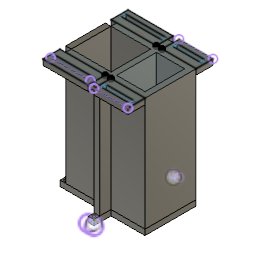
dobot_magician_holder_210mm (Autodesk Fusion 360 design; units mm, degrees)
Autodesk Fusion 360 part; units mm, degrees
note: some values were not read from the file. Chosen so that the rebuilt part matches the saved one: which bodies a step acts on.
sketch "スケッチ1" plane through (0, 0, 0) normal (0, 0, 1) x (1, 0, 0)
  line L0 (5, 75) -> (-5, 75)
  line L1 (-5, 75) -> (-5, -75)
  line L2 (-5, -75) -> (5, -75)
  line L3 (5, -75) -> (5, 75)
  line L4 (5, 75) -> (-5, -75) construction
  line L5 (-5, 75) -> (5, -75) construction
  dimension "d1" = 10
  dimension "d2" = 150
  constraint horizontal L0
  constraint perpendicular L0 L1
  constraint parallel L0 L2
  constraint parallel L1 L3
  constraint coincident L4 origin
  constraint coincident L5 origin
  measures "d1" distance of L1.end L2.end
  measures "d2" distance of L0.end L1.end
sketch "スケッチ2" plane through (0, 0, 0) normal (0, 0, 1) x (1, 0, 0)
  circle A0 centre (0, 70) radius 2.5
  line L0 (5, 75) -> (-5, 75)
  circle A1 centre (0, -70) radius 2.5
  line L1 (-5, -75) -> (5, -75)
  dimension "d3" = 5
  dimension "d4" = 5
  dimension "d5" = 5
  dimension "d6" = 5
  measures "d3" diameter of A0
  measures "d4" distance of A0.centre L0
  measures "d5" diameter of A1
  measures "d6" distance of A1.centre L1
extrude "押し出し1" add sketch "スケッチ1" along normal blind 1 makes body 1
extrude "押し出し2" cut sketch "スケッチ2" along normal blind 2 contours A1 bodies 1
sketch "スケッチ3" plane through (0, 0, 0) normal (0, 0, 1) x (1, 0, 0)
  line L0 (-75, 45) -> (-85, 45)
  line L1 (-85, 45) -> (-85, -45)
  line L2 (-85, -45) -> (-75, -45)
  line L3 (-75, -45) -> (-75, 45)
  line L4 (-75, 45) -> (-85, -45) construction
  line L5 (-85, 45) -> (-75, -45) construction
  circle A0 centre (-80, 40) radius 2.5
  circle A1 centre (-80, -40) radius 2.5
  line L6 (-85, 45) -> (65, 45)
  line L7 (65, 45) -> (65, 35)
  line L8 (65, 35) -> (-85, 35)
  line L9 (-85, 35) -> (-85, 45)
  line L10 (-85, -45) -> (65, -45)
  line L11 (65, -45) -> (65, -35)
  line L12 (65, -35) -> (-85, -35)
  line L13 (-85, -35) -> (-85, -45)
  line L14 (55, 45) -> (65, 45)
  line L15 (65, 45) -> (65, -45)
  line L16 (65, -45) -> (55, -45)
  line L17 (55, -45) -> (55, 45)
  point P0 (-80, 0)
  point P1 (0, 70)
  dimension "d11" = 10
  dimension "d12" = 90
  dimension "d13" = 5
  dimension "d14" = 5
  dimension "d15" = 80
  dimension "d16" = 5
  dimension "d17" = 5
  dimension "d18" = 150
  dimension "d19" = 10
  dimension "d20" = 150
  dimension "d21" = 10
  constraint horizontal L0
  constraint perpendicular L0 L1
  constraint parallel L0 L2
  constraint parallel L1 L3
  constraint coincident L4 P0
  constraint coincident L5 P0
  constraint horizontal L6
  constraint vertical L7
  constraint horizontal L8
  constraint vertical L9
  constraint horizontal L10
  constraint vertical L11
  constraint horizontal L12
  constraint vertical L13
  constraint horizontal L14
  constraint vertical L15
  constraint horizontal L16
  constraint vertical L17
  constraint coincident L6 L14.start
  measures "d11" distance of L1.end L2.end
  measures "d12" distance of L0.end L1.end
  measures "d13" diameter of A0
  measures "d14" diameter of A1
  measures "d15" horizontal distance of A0.centre P1
  measures "d16" distance of L1 A0.centre
  measures "d17" distance of L1 A1.centre
  measures "d18" distance of L0.end L6.end
  measures "d19" distance of L0.end L8.end
  measures "d20" distance of L1.end L10.end
  measures "d21" distance of L1.end L12.end
extrude "押し出し3" add sketch "スケッチ3" along normal blind 1 contours L0 L1 L3 L6 L8 L9 | L3 L6 L8 L17 | L1 L3 L8 L12 | L6 L7 L8 L14 L15 L17 | L3 L10 L12 L17 | L1 L2 L3 L10 L12 L13 | L8 L12 L15 L17 | L10 L11 L12 L15 L16 L17 bodies 1
extrude "押し出し4" cut sketch "スケッチ2" along normal blind 2 contours A0 bodies 1
fillet "フィレット1" radius 1 1 faces at (61.6667, -11.6667, 0) on bodies 1
extrude "押し出し5" add 1 faces at (61.6667, -11.6667, 1) along direction (0, 0, 1) blind 10 on bodies 1 bodies 1
sketch "スケッチ4" plane through (0, 0, 11) normal (0, 0, 1) x (-1, 0, 0)
  circle A0 centre (0, -70) radius 2.5
  line L0 (5, -35) -> (5, 35)
  line L1 (5, 35) -> (75, 35)
  line L2 (75, 35) -> (75, -35)
  line L3 (75, -35) -> (5, -35)
  line L4 (5, -45) -> (85, -45)
  line L5 (85, -45) -> (85, 45)
  line L6 (85, 45) -> (5, 45)
  line L7 (5, 45) -> (5, 75)
  line L8 (5, 75) -> (-5, 75)
  line L9 (-5, 75) -> (-5, 45)
  line L10 (-5, 45) -> (-65, 45)
  line L11 (-65, 45) -> (-65, -45)
  line L12 (-65, -45) -> (-5, -45)
  line L13 (-5, -45) -> (-5, -75)
  line L14 (-5, -75) -> (5, -75)
  line L15 (5, -75) -> (5, -45)
  circle A1 centre (80, 40) radius 2.5
  circle A2 centre (80, -40) radius 2.5
  circle A3 centre (0, 70) radius 2.5
  line L16 (-5, -35) -> (-55, -35)
  line L17 (-55, -35) -> (-55, 35)
  line L18 (-55, 35) -> (-5, 35)
  line L19 (-5, 35) -> (-5, -35)
  line L20 (75, -45) -> (-65, -45)
  line L21 (-65, -45) -> (-65, -35)
  line L22 (-65, -35) -> (75, -35)
  line L23 (75, -35) -> (75, -45)
  line L24 (75, 35) -> (-65, 35)
  line L25 (-65, 35) -> (-65, 45)
  line L26 (-65, 45) -> (75, 45)
  line L27 (75, 45) -> (75, 35)
  line L28 (-65, 35) -> (-55, 35)
  line L29 (-55, 35) -> (-55, -35)
  line L30 (-55, -35) -> (-65, -35)
  line L31 (-65, -35) -> (-65, 35)
  line L32 (75, -35) -> (85, -35)
  line L33 (85, -35) -> (85, 35)
  line L34 (85, 35) -> (75, 35)
  line L35 (75, 35) -> (75, -35)
  line L36 (5, -65) -> (-5, -65)
  line L37 (-5, -65) -> (-5, 65)
  line L38 (-5, 65) -> (5, 65)
  line L39 (5, 65) -> (5, -65)
  constraint horizontal L20
  constraint vertical L21
  constraint horizontal L22
  constraint vertical L23
  constraint coincident L11 L21.end
  constraint coincident L4 L20.start
  constraint horizontal L24
  constraint vertical L25
  constraint horizontal L26
  constraint vertical L27
  constraint coincident L10.end L11.start
  constraint coincident L1.end L2.start
  constraint horizontal L28
  constraint vertical L29
  constraint horizontal L30
  constraint vertical L31
  constraint coincident L16.end L17.start
  constraint horizontal L32
  constraint vertical L33
  constraint horizontal L34
  constraint vertical L35
  constraint coincident L5 L33.end
  constraint horizontal L36
  constraint vertical L37
  constraint horizontal L38
  constraint vertical L39
  constraint coincident L9 L37.end
  constraint coincident L15 L36.start
extrude "押し出し6" add sketch "スケッチ4" along normal blind 200 separate body contours L0 L19 L22 L24 L37 L39 | L20 L22 L37 L39 | L3 L4 L20 L22 L23 L39 | L1 L6 L24 L26 L27 L39 | L24 L26 L37 L39 | L2 L5 L32 L33 L34 L35 | L11 L12 L16 L20 L21 L22 L30 L37 | L13 L15 L20 L36 L37 L39 | L10 L11 L18 L24 L25 L26 L28 L37 | L7 L9 L26 L37 L38 L39 | L11 L17 L22 L24 L28 L29 L30 L31 makes body 2 at (-75, -11.6667, 77.6667)
sketch "スケッチ5" plane through (0, 0, 211) normal (0, 0, 1) x (-1, 0, 0)
  line L0 (-5, -35) -> (-55, -35)
  line L1 (-55, -35) -> (-55, 35)
  line L2 (-55, 35) -> (-5, 35)
  line L3 (-5, 35) -> (-5, -35)
  line L4 (5, 65) -> (-5, 65)
  line L5 (-5, 65) -> (-5, 45)
  line L6 (-5, 45) -> (-65, 45)
  line L7 (-65, 45) -> (-65, -45)
  line L8 (-65, -45) -> (-5, -45)
  line L9 (-5, -45) -> (-5, -65)
  line L10 (-5, -65) -> (5, -65)
  line L11 (5, -65) -> (5, -45)
  line L12 (5, -45) -> (75, -45)
  line L13 (75, -45) -> (75, -35)
  line L14 (75, -35) -> (5, -35)
  line L15 (5, -35) -> (5, 35)
  line L16 (5, 35) -> (75, 35)
  line L17 (75, 35) -> (75, 45)
  line L18 (75, 45) -> (5, 45)
  line L19 (5, 45) -> (5, 65)
  line L20 (5, 45) -> (85, 45)
  line L21 (85, 45) -> (85, 75)
  line L22 (85, 75) -> (5, 75)
  line L23 (5, 75) -> (5, 45)
  line L24 (-5, 45) -> (-65, 45)
  line L25 (-65, 45) -> (-65, 75)
  line L26 (-65, 75) -> (-5, 75)
  line L27 (-5, 75) -> (-5, 45)
  line L28 (5, -45) -> (85, -45)
  line L29 (85, -45) -> (85, -75)
  line L30 (85, -75) -> (5, -75)
  line L31 (5, -75) -> (5, -45)
  line L32 (-5, -45) -> (-65, -45)
  line L33 (-65, -45) -> (-65, -75)
  line L34 (-65, -75) -> (-5, -75)
  line L35 (-5, -75) -> (-5, -45)
  line L36 (80, -66.5) -> (10, -66.5)
  line L37 (10, -66.5) -> (10, -58.5)
  line L38 (10, -58.5) -> (80, -58.5)
  line L39 (80, -58.5) -> (80, -66.5)
  line L40 (80, 58.5) -> (10, 58.5)
  line L41 (10, 58.5) -> (10, 66.5)
  line L42 (10, 66.5) -> (80, 66.5)
  line L43 (80, 66.5) -> (80, 58.5)
  dimension "d32" = 80
  dimension "d33" = 30
  dimension "d34" = 60
  dimension "d35" = 30
  dimension "d36" = 80
  dimension "d37" = 30
  dimension "d38" = 60
  dimension "d39" = 30
  dimension "d42" = 8.5
  dimension "d52" = 8
  dimension "d53" = 8.5
  dimension "d54" = 8
  constraint horizontal L20
  constraint vertical L21
  constraint horizontal L22
  constraint vertical L23
  constraint coincident L18.end L19.start
  constraint horizontal L24
  constraint vertical L25
  constraint horizontal L26
  constraint vertical L27
  constraint coincident L5.end L6.start
  constraint horizontal L28
  constraint vertical L29
  constraint horizontal L30
  constraint vertical L31
  constraint coincident L11.end L12.start
  constraint horizontal L32
  constraint vertical L33
  constraint horizontal L34
  constraint vertical L35
  constraint coincident L8.end L9.start
  constraint horizontal L36
  constraint vertical L37
  constraint horizontal L38
  constraint vertical L39
  constraint horizontal L40
  constraint vertical L41
  constraint horizontal L42
  constraint vertical L43
  measures "d32" distance of L18.end L20.end
  measures "d33" distance of L18.end L22.end
  measures "d34" distance of L5.end L6.end
  measures "d35" distance of L5.end L26.end
  measures "d36" distance of L11.end L28.end
  measures "d37" distance of L11.end L30.end
  measures "d38" distance of L8.end L7.end
  measures "d39" distance of L8.end L34.end
  measures "d42" distance of L30 L36
  measures "d52" distance of L36 L38
  measures "d53" distance of L22 L42
  measures "d54" distance of L40 L42
sketch "スケッチ6" plane through (0, 0, 211) normal (0, 0, 1) x (1, 0, 0)
sketch "スケッチ7" plane through (0, 0, 51) normal (0, 0, 1) x (-1, 0, 0)
sketch "スケッチ8" plane through (0, 0, 211) normal (0, 0, 1) x (-1, 0, 0)
  line L0 (-9.8252, -66.5) -> (-59.8252, -66.5)
  line L1 (-59.8252, -66.5) -> (-59.8252, -58.5)
  line L2 (-59.8252, -58.5) -> (-9.8252, -58.5)
  line L3 (-9.8252, -58.5) -> (-9.8252, -66.5)
  line L4 (-65, -75) -> (-5, -75)
  line L5 (-10, 66.5) -> (-60, 66.5)
  line L6 (-60, 66.5) -> (-60, 58.5)
  line L7 (-60, 58.5) -> (-10, 58.5)
  line L8 (-10, 58.5) -> (-10, 66.5)
  line L9 (10, 66.5) -> (80, 66.5)
  line L10 (-65, 75) -> (-5, 75)
  dimension "d43" = 50
  dimension "d44" = 8
  dimension "d45" = 8.5
  dimension "d50" = 8
  dimension "d51" = 8.5
  constraint horizontal L0
  constraint vertical L1
  constraint horizontal L2
  constraint vertical L3
  constraint horizontal L5
  constraint vertical L6
  constraint vertical L8
  measures "d43" distance of L0.start L0.end
  measures "d44" distance of L0.start L2.end
  measures "d45" distance of L0 L4
  measures "d50" distance of L5 L7
  measures "d51" distance of L5 L10
extrude "押し出し7" add sketch "スケッチ5" against normal blind 10 separate body contours L18 L19 L20 L21 L22 L23 | L5 L6 L24 L25 L26 L27 | L8 L9 L32 L33 L34 L35 | L11 L12 L28 L29 L30 L31 makes body 3 at (45, -65, 211) makes body 4 at (-56.6667, -49.5, 211) makes body 5 at (-33.3333, 49.5, 211) makes body 6 at (45, 65, 211)
extrude "押し出し8" cut sketch "スケッチ8" against normal blind 10 bodies 3 6
